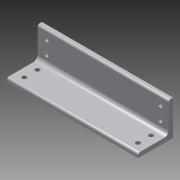
# Autodesk Inventor part: Right Angle
Saved by Autodesk Inventor 2016 (Build 200138000, 138)
## iProperties
Created: 2016-04-02
Part Number: Right Angle
Material: Aluminum 6061
Document SubType Name: Modeling
Designer: hwasserb
Density: 2.71 g/cm^3
Appearance: Aluminum - Flat
Author: hwasserb
Autodesk Inventor part; units mm, degrees
ref_plane "YZ Plane" through (0, 0, 0) normal (1, 0, 0) x (0, 1, 0)
ref_plane "XZ Plane" through (0, 0, 0) normal (0, 1, 0) x (-1, 0, 0)
ref_plane "XY Plane" through (0, 0, 0) normal (0, 0, 1) x (1, 0, 0)
sketch "Sketch1" plane through (0, 0, 0) normal (0, 0, 1) x (1, 0, 0)
  line L0 (0, 0) -> (50.8, 0)
  line L1 (50.8, 0) -> (50.8, 50.8)
  line L2 (50.8, 50.8) -> (47.625, 50.8)
  line L3 (44.45, 47.625) -> (44.45, 12.7)
  line L4 (38.1, 6.35) -> (3.175, 6.35)
  line L5 (0, 3.175) -> (0, 0)
  arc A0 (3.175, 6.35) -> (0, 3.175) centre (3.175, 3.175) ccw
  arc A1 (47.625, 50.8) -> (44.45, 47.625) centre (47.625, 47.625) ccw
  arc A2 (38.1, 6.35) -> (44.45, 12.7) centre (38.1, 12.7) ccw
  dimension "d0" = 50.8
  dimension "d1" = 6.35
  dimension "d2" = 3.175
  dimension "d3" = 6.35
  constraints: 12 end point, 6 point on circle, 6 tangent, 4 parallel, 3 centre point, 3 perpendicular, 1 equal radius, 1 horizontal
  measures "d0" distance of L0.start L0.end
  measures "d1" distance between parallel lines of L0 L4
  measures "d2" radius of A0
  measures "d3" radius of A2
extrude "Extrusion1" add sketch "Sketch1" along normal blind 190.5
sketch "Sketch2" plane through (0, 0, 0) normal (0, -1, 0) x (1, 0, 0)
  line L0 (0, 0) -> (50.8, 0) projected
  line L1 (0, 190.5) -> (50.8, 190.5) projected
  line L2 (0, 0) -> (0, 190.5) projected
  point P0 (12.7, 177.8)
  point P1 (31.75, 177.8)
  point P2 (12.7, 12.7)
  point P3 (31.75, 12.7)
  dimension "d6" = 19.05
  dimension "d7" = 12.7
  dimension "d8" = 12.7
  dimension "d9" = 12.7
  constraints: 2 horizontal alignment, 2 vertical alignment
  measures "d6" distance of point (31.75, 177.8) point (12.7, 177.8)
  measures "d7" distance from line of L1 point (12.7, 177.8)
  measures "d8" distance from line of L0 point (12.7, 12.7)
  measures "d9" distance from line of point (12.7, 12.7) L2
hole "Hole1" at (12.7, 0, 177.8) at (31.75, 0, 177.8) at (12.7, 0, 12.7) at (31.75, 0, 12.7) direction (0, 1, 0) diameter 6.35 end through all
sketch "Sketch3" plane through (50.8, 0, 0) normal (1, 0, 0) x (0, 0, -1)
  line L0 (0, 0) -> (0, 50.8) projected
  line L1 (0, 50.8) -> (-190.5, 50.8) projected
  line L2 (-190.5, 0) -> (-190.5, 50.8) projected
  point P0 (-177.8, 19.05)
  point P1 (-177.8, 38.1)
  point P2 (-12.7, 19.05)
  point P3 (-12.7, 38.1)
  dimension "d17" = 19.05
  dimension "d18" = 12.7
  dimension "d19" = 12.7
  dimension "d20" = 12.7
  constraints: 2 horizontal alignment, 2 vertical alignment
  measures "d17" distance of point (-177.8, 19.05) point (-177.8, 38.1)
  measures "d18" distance from line of L2 point (-177.8, 38.1)
  measures "d19" distance from line of L1 point (-177.8, 38.1)
  measures "d20" distance from line of L0 point (-12.7, 38.1)
hole "Hole2" at (50.8, 19.05, 177.8) at (50.8, 38.1, 177.8) at (50.8, 19.05, 12.7) at (50.8, 38.1, 12.7) direction (-1, 0, 0) diameter 6.35 end through all
body "Solid1"
